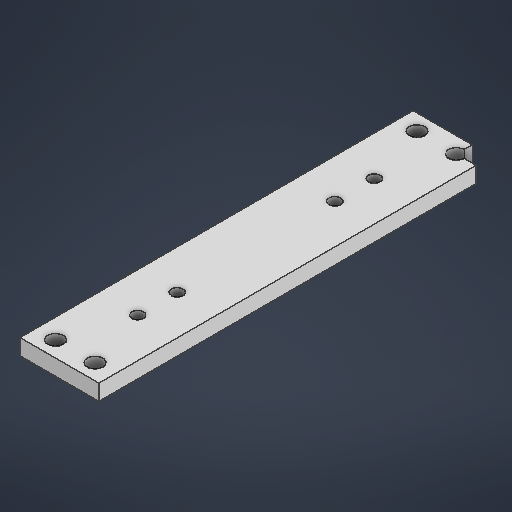
# Autodesk Inventor part: side_wall1
Saved by Autodesk Inventor 2026.1 (Build 301233000, 233)
## iProperties
Created: 2026-03-24
Part Number: side_wall1
Material: Generic
Document SubType Name: Modeling
Designer: emanuel
Density: 1 g/cm^3
Appearance: Default
Author: emanuel
Autodesk Inventor part; units mm, degrees
ref_plane "YZ Plane" through (0, 0, 0) normal (1, 0, 0) x (0, 1, 0)
ref_plane "XZ Plane" through (0, 0, 0) normal (0, 1, 0) x (-1, 0, 0)
ref_plane "XY Plane" through (0, 0, 0) normal (0, 0, 1) x (1, 0, 0)
sketch "Sketch1" plane through (0, 0, 0) normal (0, 1, 0) x (-1, 0, 0)
  line L0 (0, 0) -> (10, 0)
  line L1 (10, 0) -> (10, -91.7)
  line L2 (10, -91.7) -> (0, -91.7)
  line L3 (0, -91.7) -> (0, 0)
  circle A0 centre (10, 0) radius 2
  circle A1 centre (0, 0) radius 2
  circle A2 centre (10, -91.7) radius 2
  circle A3 centre (0, -91.7) radius 2
  line L4 (10, 0) -> (15, 0)
  line L5 (15, 0) -> (15, 4)
  line L6 (15, 4) -> (10, 4)
  line L7 (10, 4) -> (10, 0)
  line L8 (0, -91.7) -> (-5, -91.7)
  line L9 (-5, -91.7) -> (-5, -95.7)
  line L10 (-5, -95.7) -> (0, -95.7)
  line L11 (0, -95.7) -> (0, -91.7)
  line L12 (15, 4) -> (-5, 4)
  line L13 (-5, 4) -> (-5, -95.7)
  line L14 (-5, -95.7) -> (15, -95.7)
  line L15 (15, -95.7) -> (15, 4)
  line L16 (5, 0) -> (5, -91.7)
  line L17 (5, -20.85) -> (5, -70.85)
  line L18 (5, -15.85) -> (5, -25.85)
  line L19 (5, -65.85) -> (5, -75.85)
  circle A4 centre (5, -15.85) radius 1.5
  circle A5 centre (5, -25.85) radius 1.5
  circle A6 centre (5, -65.85) radius 1.5
  circle A7 centre (5, -75.85) radius 1.5
  point P0 (5, -45.85)
  point P1 (-2, -91.7)
  point P2 (0, -93.7)
  dimension "d0" = 10
  dimension "d1" = 91.7
  dimension "d2" = 4
  dimension "d3" = 4
  dimension "d4" = 4
  dimension "d5" = 4
  dimension "d6" = 5
  dimension "d7" = 4
  dimension "d8" = 5
  dimension "d9" = 4
  dimension "d10" = 50
  dimension "d11" = 10
  dimension "d12" = 10
  dimension "d13" = 3
  dimension "d14" = 3
  dimension "d15" = 3
  dimension "d16" = 3
  constraints: 40 end point, 8 centre point, 8 coincident, 8 parallel, 6 midpoint, 4 horizontal, 4 perpendicular, 3 point on line
  measures "d0" distance of L1.end L2.end
  measures "d1" distance of L0.end L1.end
  measures "d2" diameter of A0
  measures "d3" diameter of A1
  measures "d4" diameter of A2
  measures "d5" diameter of A3
  measures "d6" distance of L6.end L5.end
  measures "d7" distance of L5.end L4.end
  measures "d8" distance of L10.end L9.end
  measures "d9" distance of L9.end L8.end
  measures "d10" distance of L17.start L17.end
  measures "d11" distance of L18.start L18.end
  measures "d12" distance of L19.start L19.end
  measures "d13" diameter of A4
  measures "d14" diameter of A5
  measures "d15" diameter of A6
  measures "d16" diameter of A7
extrude "Extrusion1" add sketch "Sketch1" along normal blind 4 contours A1 L3 A3 L8 L13 L12 L7 A0 L0 | L0 L16 A4 A5 A6 A7 L2 A3 L3 A1 | L0 A0 L1 A2 L2 L16 A7 A6 A5 A4 | L2 A2 L1 A0 L4 L15 L14 L11 A3 | L7 L6 L5 L4 A0
body "Solid1"
